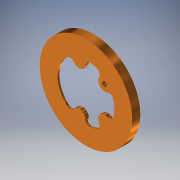
# Autodesk Inventor part: Ring Holder
Saved by Autodesk Inventor 2017 (Build 210142000, 142)
## iProperties
Created: 2017-01-05
Part Number: Ring Holder
Material: Gold
Document SubType Name: Modeling
Designer: PLTW
Density: 19.3 g/cm^3
Appearance: Metal 1600F Hot
Author: PLTW
Autodesk Inventor part; units mm, degrees
ref_plane "YZ Plane" through (0, 0, 0) normal (1, 0, 0) x (0, 1, 0)
ref_plane "XZ Plane" through (0, 0, 0) normal (0, 1, 0) x (-1, 0, 0)
ref_plane "Work Plane1" through (0, 23.1367, 0) normal (0, 0, 1) x (1, 0, 0)
sketch "Sketch1" plane through (0, 23.1367, 0) normal (0, 0, 1) x (1, 0, 0)
  circle A0 centre (0, 0) radius 1.905 projected
  circle A1 centre (0, 0) radius 4.318 projected
  circle A2 centre (0, -23.1367) radius 4.318 projected
  circle A3 centre (-17.907, -28.3507) radius 1.905 projected
  circle A4 centre (-17.907, -28.3507) radius 4.318 projected
  circle A5 centre (-17.907, 5.2141) radius 1.905 projected
  circle A6 centre (-17.907, 5.2141) radius 4.318 projected
  circle A7 centre (0, -23.1367) radius 1.905 projected
  point P0 (0, -23.1367)
extrude "Extrusion1" add sketch "Sketch1" along normal blind 1.27
sketch "Sketch2" plane through (0, 23.1367, 1.27) normal (0, 0, 1) x (1, 0, 0)
  circle A0 centre (0, 0) radius 1.905 projected
  circle A1 centre (-13.081, -11.5683) radius 29.972 construction
  circle A2 centre (0, -23.1367) radius 4.318 projected
  circle A3 centre (-17.907, -28.3507) radius 4.318 projected
  circle A4 centre (-17.907, 5.2141) radius 4.318 projected
  circle A5 centre (0, 0) radius 4.318 projected
  arc A6 (-26.3706, 3.3811) -> (-26.3706, -26.5178) centre (-13.081, -11.5683) ccw projected
  arc A7 (-21.6136, 2.7606) -> (-26.3706, 3.3811) centre (-24.2611, 1.0082) ccw projected
  arc A8 (-21.6136, 2.7606) -> (-13.4634, 5.1043) centre (-17.907, 5.2141) ccw projected
  arc A9 (-9.7626, 8.157) -> (-13.4634, 5.1043) centre (-10.2893, 5.026) ccw projected
  arc A10 (-5.2915, 6.8551) -> (-9.7626, 8.157) centre (-13.081, -11.5683) ccw projected
  arc A11 (-3.8079, 2.2929) -> (-5.2915, 6.8551) centre (-6.5279, 3.9308) ccw projected
  arc A12 (-3.8079, 2.2929) -> (1.8101, -4.0597) centre (0, 0) ccw projected
  arc A13 (6.1567, -6.09) -> (1.8101, -4.0597) centre (3.1031, -6.9596) ccw projected
  arc A14 (6.1567, -17.0467) -> (6.1567, -6.09) centre (-13.081, -11.5683) ccw projected
  arc A15 (1.8101, -19.0769) -> (6.1567, -17.0467) centre (3.1031, -16.1771) ccw projected
  arc A16 (1.8101, -19.0769) -> (-3.8079, -25.4296) centre (0, -23.1367) ccw projected
  arc A17 (-5.2915, -29.9918) -> (-3.8079, -25.4296) centre (-6.5279, -27.0674) ccw projected
  arc A18 (-9.7626, -31.2937) -> (-5.2915, -29.9918) centre (-13.081, -11.5683) ccw projected
  arc A19 (-13.4634, -28.241) -> (-9.7626, -31.2937) centre (-10.2893, -28.1626) ccw projected
  arc A20 (-13.4634, -28.241) -> (-21.6136, -25.8973) centre (-17.907, -28.3507) ccw projected
  arc A21 (-26.3706, -26.5178) -> (-21.6136, -25.8973) centre (-24.2611, -24.1449) ccw projected
  circle A22 centre (-13.081, -11.5683) radius 23.1775 construction
  circle A23 centre (-13.081, -11.5683) radius 32.639
  circle A24 centre (-17.907, 5.2141) radius 1.905 projected
  circle A25 centre (-17.907, -28.3507) radius 1.905 projected
  circle A26 centre (0, -23.1367) radius 1.905 projected
  point P0 (0, -23.1367)
  dimension "d2" = 2.667
  constraints: 1 centre point, 1 concentric
  measures "d2" radial gap between concentric circles of A1 A23
extrude "Extrusion2" add sketch "Sketch2" along normal blind 1.27 contours A2 | A3 | A4 | A5 | A23
sketch "Sketch3" plane through (-13.081, 11.5683, 1.27) normal (0, 0, -1) x (-1, 0, 0)
  circle A0 centre (0, 0) radius 32.639 projected
  circle A1 centre (0, 0) radius 30.226
  circle A2 centre (0, 0) radius 29.972 construction
  dimension "d5" = 0.254
  constraints: 1 centre point, 1 coincident
  measures "d5" radial gap between concentric circles of A2 A1
extrude "Extrusion3" add sketch "Sketch3" along normal blind 4.445
sketch "Sketch4" plane through (-13.081, 11.5683, 2.54) normal (0, 0, 1) x (1, 0, 0)
  circle A0 centre (0, 0) radius 32.639 projected
  line L0 (-25.7884, 14.4733) -> (-19.6831, 10.5838) projected
  line L1 (-23.9803, 13.3214) -> (-21.297, 11.612) projected
  line L2 (-20.6583, 8.8945) -> (-27.0794, 12.2371) projected
  arc A1 (-19.6831, 10.5838) -> (-20.6583, 8.8945) centre (-0.8255, -1.4298) ccw projected
  arc A2 (-25.7884, 14.4733) -> (-27.0794, 12.2371) centre (-0.8255, -1.4298) ccw projected
  line L3 (-13.6447, 9.7608) -> (-30.5534, 18.3036)
  line L4 (-30.5534, 18.3036) -> (-32.8613, 13.7354)
  line L5 (-32.8613, 13.7354) -> (-15.9527, 5.1927)
  line L6 (-15.9527, 5.1927) -> (-13.6447, 9.7608)
  line L7 (-13.6447, 9.7608) -> (-32.8613, 13.7354) construction
  line L8 (-30.5534, 18.3036) -> (-15.9527, 5.1927) construction
  line L9 (0, 0) -> (-35.2926, 17.8309) construction
  point P0 (-23.253, 11.7481)
  point P1 (-23.253, 11.7481)
  dimension "d8" = 1.27
  dimension "d9" = 1.27
  constraints: 14 end point, 3 midpoint, 2 parallel, 2 perpendicular, 1 point on line
  measures "d8" distance from line of L3 L0.start
  measures "d9" distance from line of L5 L2.end
ref_plane "Work Plane2" through (-43.053, -18.4037, -2.159) normal (0, 0, -1) x (0, 1, 0)
extrude "Extrusion4" cut sketch "Sketch4" against normal up to surface (4.699 mm away) contours L3 L6 L5 A0 | A0 L5 L4 L3 | L0 A1 L2 A2 picked at (-16.4268, 8.5124)
fillet "Fillet1" radius 2.54 2 edges at (-42.1969, 23.4114, -2.159) (-39.8889, 27.9796, -2.159)
equation "\"d9\" = d8"
body "Solid1"
